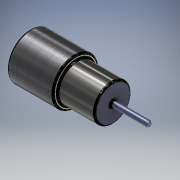
# Autodesk Inventor part: 马达
Saved by Autodesk Inventor 2017 (Build 210142000, 142)
## iProperties
Part Number: 马达
Material: 常规
Document SubType Name: Modeling
Designer: PANDA
Density: 1 g/cm^3
Appearance: 默认
Author: PANDA
Autodesk Inventor part; units mm, degrees
ref_plane "YZ Plane" through (0, 0, 0) normal (1, 0, 0) x (0, 1, 0)
ref_plane "XZ Plane" through (0, 0, 0) normal (0, 1, 0) x (-1, 0, 0)
ref_plane "XY Plane" through (0, 0, 0) normal (0, 0, 1) x (1, 0, 0)
sketch "草图1" plane through (0, 0, 0) normal (1, 0, 0) x (0, 1, 0)
  circle A0 centre (0, 0) radius 25
  dimension "d0" = 50
  constraints: 1 centre point, 1 coincident
  measures "d0" diameter of A0
extrude "拉伸1" add sketch "草图1" along normal blind 50
sketch "草图2" plane through (50, 0, 0) normal (1, 0, 0) x (0, 0, -1)
  circle A0 centre (0, 0) radius 20
  dimension "d3" = 40
  constraints: 1 centre point, 1 coincident
  measures "d3" diameter of A0
extrude "拉伸2" add sketch "草图2" along normal blind 40
sketch "草图3" plane through (90, 0, 0) normal (1, 0, 0) x (0, 0, -1)
  circle A0 centre (0, 0) radius 3
  dimension "d6" = 6
  constraints: 1 centre point, 1 coincident
  measures "d6" diameter of A0
extrude "拉伸3" add sketch "草图3" along normal blind 40
fillet "圆角1" radius 2 1 edges at (130, 0, 3)
fillet "圆角2" radius 2 1 edges at (90, 0, 20)
fillet "圆角3" radius 2 2 edges at (50, -25, 0) (0, -25, 0)
fillet "圆角3" radius 2 2 edges at (90, 0, 3) (50, 0, 20)
